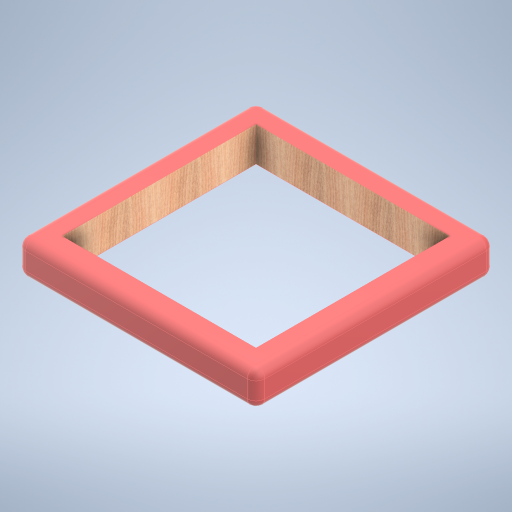
# Autodesk Inventor part: Bumpers
Saved by Autodesk Inventor 2024.2 (Build 282272000, 272)
## iProperties
Created: 2024-01-14
Part Number: Bumpers
Material: Generic
Document SubType Name: Modeling
Designer: rohan
Density: 1 g/cm^3
Appearance: Smooth - Red
RuleStatus: InUse
AfterAnyParamChange0: Bumper_Measurements
AfterAnyParamChange1: Bumper_Suppression
AfterAnyUserParamChange0: Bumper_Measurements
AfterAnyUserParamChange1: Bumper_Suppression
AfterFeatureSuppressionChange0: Bumper_Measurements
AfterFeatureSuppressionChange1: Bumper_Suppression
PartBodyChanged0: Bumper_Measurements
PartBodyChanged1: Bumper_Suppression
Author: rohan
Autodesk Inventor part; units mm, degrees
ref_plane "YZ Plane" through (0, 0, 0) normal (1, 0, 0) x (0, 1, 0)
ref_plane "XZ Plane" through (0, 0, 0) normal (0, 1, 0) x (-1, 0, 0)
ref_plane "XY Plane" through (0, 0, 0) normal (0, 0, 1) x (1, 0, 0)
sketch "Sketch1" plane through (0, 0, 0) normal (0, 1, 0) x (-1, 0, 0)
  line L0 (355.6, 355.6) -> (-355.6, 355.6)
  line L1 (-355.6, 355.6) -> (-355.6, -355.6)
  line L2 (-355.6, -355.6) -> (355.6, -355.6)
  line L3 (355.6, -355.6) -> (355.6, 355.6)
  line L4 (355.6, 355.6) -> (-355.6, -355.6) construction
  line L5 (-355.6, 355.6) -> (355.6, -355.6) construction
  line L6 (438.15, 438.15) -> (-438.15, 438.15)
  line L7 (-438.15, 438.15) -> (-438.15, -438.15)
  line L8 (-438.15, -438.15) -> (438.15, -438.15)
  line L9 (438.15, -438.15) -> (438.15, 438.15)
  line L10 (438.15, 438.15) -> (-438.15, -438.15) construction
  line L11 (-438.15, 438.15) -> (438.15, -438.15) construction
  point P0 (0, 0)
  dimension "d0" = 82.55
  dimension "d1" = 82.55
  dimension "d2" = 711.2
  dimension "d3" = 711.2
  constraints: 24 end point, 4 midpoint, 4 parallel, 2 horizontal, 2 perpendicular
  measures "d0" distance between parallel lines of L2 L8
  measures "d1" distance between parallel lines of L3 L9
  measures "d2" distance of L2.end L0.start
  measures "d3" distance of L0.start L0.end
extrude "Extrusion1" add sketch "Sketch1" along normal blind 127
fillet "Fillet1" radius 31.75 12 edges at (0, 127, 438.15) (0, 0, 438.15) (438.15, 63.5, 438.15) (438.15, 127, 0) (438.15, 0, 0) (438.15, 63.5, -438.15) (0, 127, -438.15) (-438.15, 127, 0) (-438.15, 63.5, 438.15) (0, 0, -438.15) (-438.15, 63.5, -438.15) (-438.15, 0, 0)
sketch "Bumper_Gaps" plane through (0, 127, 0) normal (0, 1, 0) x (1, 0, 0)
  line L0 (-203.2, -438.15) -> (203.2, -438.15)
  line L1 (203.2, -438.15) -> (203.2, -355.6)
  line L2 (203.2, -355.6) -> (-203.2, -355.6)
  line L3 (-203.2, -355.6) -> (-203.2, -438.15)
  line L4 (-203.2, -438.15) -> (203.2, -355.6) construction
  line L5 (203.2, -438.15) -> (-203.2, -355.6) construction
  line L6 (-438.15, -254) -> (-355.6, -254)
  line L7 (-355.6, -254) -> (-355.6, 254)
  line L8 (-355.6, 254) -> (-438.15, 254)
  line L9 (-438.15, 254) -> (-438.15, -254)
  line L10 (-438.15, -254) -> (-355.6, 254) construction
  line L11 (-355.6, -254) -> (-438.15, 254) construction
  line L12 (355.6, -254) -> (438.15, -254)
  line L13 (438.15, -254) -> (438.15, 254)
  line L14 (438.15, 254) -> (355.6, 254)
  line L15 (355.6, 254) -> (355.6, -254)
  line L16 (355.6, -254) -> (438.15, 254) construction
  line L17 (438.15, -254) -> (355.6, 254) construction
  line L18 (-355.6, -355.6) -> (-355.6, 355.6) projected
  line L19 (-438.15, 406.4) -> (-438.15, -406.4) projected
  line L20 (355.6, 355.6) -> (355.6, -355.6) projected
  line L21 (438.15, -406.4) -> (438.15, 406.4) projected
  line L22 (355.6, -355.6) -> (-355.6, -355.6) projected
  line L23 (-406.4, -438.15) -> (406.4, -438.15) projected
  line L24 (-196.85, 355.6) -> (196.85, 355.6)
  line L25 (196.85, 355.6) -> (196.85, 438.15)
  line L26 (196.85, 438.15) -> (-196.85, 438.15)
  line L27 (-196.85, 438.15) -> (-196.85, 355.6)
  line L28 (-196.85, 355.6) -> (196.85, 438.15) construction
  line L29 (196.85, 355.6) -> (-196.85, 438.15) construction
  line L30 (406.4, 438.15) -> (-406.4, 438.15) projected
  line L31 (-355.6, 355.6) -> (355.6, 355.6) projected
  point P0 (0, 0)
  point P1 (0, -396.875)
  point P2 (-396.875, 0)
  point P3 (396.875, 0)
  point P4 (0, 396.875)
  dimension "d15" = 406.4
  dimension "d16" = 393.7
  dimension "d17" = 508
  dimension "d18" = 508
  constraints: 48 end point, 8 collinear, 8 midpoint, 8 parallel, 4 horizontal, 4 perpendicular, 2 horizontal alignment, 2 vertical alignment
  measures "d15" distance between parallel lines of L1 L3
  measures "d16" distance between parallel lines of L25 L27
  measures "d17" distance between parallel lines of L14 L12
  measures "d18" distance between parallel lines of L8 L6
extrude "Front_Gap" [suppressed]
extrude "Back_Gap" [suppressed]
extrude "Left_Gap" [suppressed]
extrude "Right_Gap" [suppressed]
equation "\"d1\" = d0"
equation "\"d2\" = Length"
equation "\"d3\" = Width"
equation "\"d15\" = Front_Width"
equation "\"d16\" = Back_Width"
equation "\"d17\" = Left_Width"
equation "\"d18\" = Right_Width"
equation "\"Length\" = 711.2"
equation "\"Width\" = 711.2"
equation "\"Front_Width\" = 406.4"
equation "\"Back_Width\" = 393.7"
equation "\"Left_Width\" = 508"
equation "\"Right_Width\" = 508"
equation "\"Front_Edge\" = 152.4"
equation "\"Back_Edge\" = 152.4"
equation "\"Left_Edge\" = 152.4"
equation "\"Right_Edge\" = 152.4"
equation "\"FECalc\" = -0.5 * Front_Width + 0.5 * Width"
equation "\"BECalc\" = -0.5 * Back_Width + 0.5 * Width"
equation "\"LECalc\" = -0.5 * Left_Width + 0.5 * Length"
equation "\"RECalc\" = -0.5 * Right_Width + 0.5 * Length"
equation "\"FWCalc\" = Width - 2 * Front_Edge"
equation "\"BWCalc\" = Width - 2 * Back_Edge"
equation "\"LWCalc\" = Length - 2 * Left_Edge"
equation "\"RWCalc\" = Length - 2 * Right_Edge"
body "Solid1"
